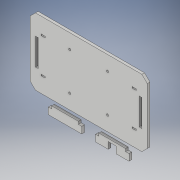
# Autodesk Inventor part: mount - developer
Saved by Autodesk Inventor 2019 (Build 230136000, 136)
## iProperties
Created: 2019-04-11
Part Number: mount - developer
Material: Generic
Document SubType Name: Modeling
Designer: jonas
Density: 1 g/cm^3
Appearance: Default
Author: jonas
Autodesk Inventor part; units mm, degrees
ref_plane "YZ Plane" through (0, 0, 0) normal (1, 0, 0) x (0, 1, 0)
ref_plane "XZ Plane" through (0, 0, 0) normal (0, 1, 0) x (-1, 0, 0)
ref_plane "XY Plane" through (0, 0, 0) normal (0, 0, 1) x (1, 0, 0)
sketch "Sketch1" plane through (0, 0, 0) normal (0, 0, 1) x (1, 0, 0)
  line L0 (-79.5, -50) -> (79.5, -50)
  line L1 (87.5, -42) -> (87.5, 42)
  line L2 (79.5, 50) -> (-79.5, 50)
  line L3 (-87.5, 42) -> (-87.5, -42)
  line L4 (0, 1.1499) -> (0, -1.1499)
  line L5 (1.5253, 0) -> (-2.0225, 0)
  line L6 (-79.5, -20) -> (-75.5, -20)
  line L7 (-75.5, -20) -> (-75.5, 20)
  line L8 (-75.5, 20) -> (-79.5, 20)
  line L9 (-79.5, 20) -> (-79.5, -20)
  line L10 (79.5, -20) -> (75.5, -20)
  line L11 (75.5, -20) -> (75.5, 20)
  line L12 (75.5, 20) -> (79.5, 20)
  line L13 (79.5, 20) -> (79.5, -20)
  line L14 (-10.2685, -72.0544) -> (-10.2685, -62.0544)
  line L15 (-10.2685, -62.0544) -> (-15.2685, -62.0544)
  line L16 (-60.2685, -62.0544) -> (-60.2685, -72.0544)
  line L17 (-60.2685, -72.0544) -> (-10.2685, -72.0544)
  line L18 (-55.2685, -58.0544) -> (-15.2685, -58.0544)
  line L19 (-15.2685, -58.0544) -> (-15.2685, -62.0544)
  line L20 (-55.2685, -62.0544) -> (-60.2685, -62.0544)
  line L21 (-55.2685, -62.0544) -> (-55.2685, -58.0544)
  circle A0 centre (-28.2843, -28.2843) radius 1.6
  circle A1 centre (28.2843, -28.2843) radius 1.6
  circle A2 centre (28.2843, 28.2843) radius 1.6
  circle A3 centre (-28.2843, 28.2843) radius 1.6
  line L22 (0, 0) -> (3.5355, -3.5355)
  line L23 (0, 0) -> (5, 0) construction
  line L24 (10.2685, -72.0544) -> (10.2685, -62.0544)
  line L25 (10.2685, -62.0544) -> (15.2685, -62.0544)
  line L26 (60.2685, -62.0544) -> (60.2685, -72.0544)
  line L27 (60.2685, -72.0544) -> (41.2685, -72.0544)
  line L28 (55.2685, -58.0544) -> (15.2685, -58.0544)
  line L29 (15.2685, -58.0544) -> (15.2685, -62.0544)
  line L30 (55.2685, -62.0544) -> (60.2685, -62.0544)
  line L31 (55.2685, -62.0544) -> (55.2685, -58.0544)
  line L32 (41.2685, -62.0544) -> (29.2685, -62.0544)
  line L33 (29.2685, -62.0544) -> (29.2685, -72.0544)
  line L34 (29.2685, -72.0544) -> (10.2685, -72.0544)
  line L35 (41.2685, -72.0544) -> (41.2685, -62.0544)
  line L36 (-71, 27) -> (-65, 27)
  line L37 (-65, 27) -> (-65, 25)
  line L38 (-65, 25) -> (-71, 25)
  line L39 (-71, 25) -> (-71, 27)
  line L40 (71, 27) -> (65, 27)
  line L41 (65, 27) -> (65, 25)
  line L42 (65, 25) -> (71, 25)
  line L43 (71, 25) -> (71, 27)
  line L44 (-71, -27) -> (-65, -27)
  line L45 (-65, -27) -> (-65, -25)
  line L46 (-65, -25) -> (-71, -25)
  line L47 (-71, -25) -> (-71, -27)
  line L48 (65, -27) -> (65, -25)
  line L49 (71, -27) -> (65, -27)
  line L50 (71, -25) -> (71, -27)
  line L51 (65, -25) -> (71, -25)
  line L52 (-79.5, 50) -> (-87.5, 42)
  line L53 (-79.5, -50) -> (-87.5, -42)
  line L54 (79.5, -50) -> (87.5, -42)
  line L55 (87.5, 42) -> (79.5, 50)
  point P0 (-87.5, -50)
  point P1 (87.5, 50)
  point P2 (87.5, -50)
  point P3 (-87.5, 50)
  dimension "d0" = 100
  dimension "d1" = 175
  dimension "d2" = 151
  dimension "d3" = 40
  dimension "d4" = 4
  dimension "d6" = 5
  dimension "d7" = 10
  dimension "d8" = 3.2
  dimension "d11" = 360
  dimension "d14" = 4
  dimension "d16" = 45
  dimension "d17" = 40
  dimension "d18" = 50
  dimension "d19" = 5
  dimension "d20" = 4
  dimension "d24" = 6
  dimension "d25" = 2
  dimension "d26" = 25
  dimension "d27" = 65
  dimension "d30" = 8
  dimension "d31" = 8
  dimension "d32" = 8
  dimension "d33" = 8
  dimension "d34" = 8
  dimension "d35" = 8
  dimension "d36" = 8
  dimension "d37" = 8
  dimension "d38" = 12
  dimension "d39" = 19
  constraints: 112 end point, 24 symmetric about line, 11 parallel, 10 point on line, 9 perpendicular, 5 horizontal, 4 centre point, 2 midpoint, 1 collinear, 1 equal length, 1 vertical, 13 other
  measures "d0" distance of point (87.5, -50) point (87.5, 50)
  measures "d1" distance of point (-87.5, -50) point (87.5, -50)
  measures "d2" distance between parallel lines of L11 L7
  measures "d3" distance of L8.end L6.start
  measures "d4" distance of L6.start L6.end
  measures "d6" distance of L14.end L15.end
  measures "d7" distance of L16.start L16.end
  measures "d8" diameter of A0
  measures "d14" distance of L20.start L18.start
  measures "d16" angle of L22 L23
  measures "d17" distance from line of A0.centre L22
  measures "d18" distance between parallel lines of L14 L16
  measures "d19" distance of L20.start L16.start
  measures "d20" distance of L18.end L15.end
  measures "d24" distance of L36.start L36.end
  measures "d25" distance of L38.end L36.start
  measures "d26" distance between parallel lines of L5 L38
  measures "d27" distance between parallel lines of L4 L37
  measures "d30" distance of L2.end point (-87.5, 50)
  measures "d31" distance of L3.start point (-87.5, 50)
  measures "d32" distance of L0.start point (-87.5, -50)
  measures "d33" distance of L3.end point (-87.5, -50)
  measures "d34" distance of L0.end point (87.5, -50)
  measures "d35" distance of L1.start point (87.5, -50)
  measures "d36" distance of L1.end point (87.5, 50)
  measures "d37" distance of L2.start point (87.5, 50)
  measures "d38" distance of L32.start L32.end
  measures "d39" distance of L33.end L24.start
extrude "Extrusion1" add sketch "Sketch1" along normal blind 4
equation "\"d14\" = d4"
equation "\"d18\" = d3 + 2 * d6"
equation "\"d31\" = d30"
equation "\"d32\" = d30"
equation "\"d33\" = d32"
equation "\"d34\" = d30"
equation "\"d35\" = d34"
equation "\"d36\" = d30"
equation "\"d37\" = d36"
body "Solid1"
